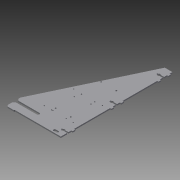
# Autodesk Inventor part: side_frame
Saved by Autodesk Inventor 2013 (Build 170138000, 138)
## iProperties
Created: 2013-11-17
Part Number: side_frame
Material: Generic
Document SubType Name: Modeling
Designer: Masta
Density: 1 g/cm^3
Author: Masta
Autodesk Inventor part; units mm, degrees
ref_plane "YZ Plane" through (0, 0, 0) normal (1, 0, 0) x (0, 1, 0)
ref_plane "XZ Plane" through (0, 0, 0) normal (0, 1, 0) x (-1, 0, 0)
ref_plane "XY Plane" through (0, 0, 0) normal (0, 0, 1) x (1, 0, 0)
sketch "Sketch1" plane through (0, 0, 0) normal (0, 0, 1) x (1, 0, 0)
  line L0 (255.7808, 350.0828) -> (255.7808, 358.8828)
  line L1 (251.6808, 67.29) -> (255.7808, 67.29)
  line L2 (255.7808, 67.29) -> (255.7808, 76.09)
  line L3 (255.7808, 76.09) -> (251.6808, 76.09)
  line L4 (251.6808, 76.09) -> (251.6808, 194.9901)
  line L5 (251.6808, 32.5401) -> (100.8808, 32.5401)
  line L6 (220.9195, 43.3685) -> (221.7479, 44.0042)
  line L7 (220.2838, 42.5401) -> (220.9195, 43.3685)
  line L8 (231.7439, 44.5401) -> (223.7479, 44.5401)
  line L9 (151.0808, 64.3506) -> (151.992, 63.6514)
  line L10 (230.5808, 213.3401) -> (234.5808, 213.3401)
  line L11 (150.0196, 64.7902) -> (151.0808, 64.3506)
  line L12 (234.5808, 211.5401) -> (239.6808, 211.5401)
  line L13 (233.7439, 44.0042) -> (234.5723, 43.3685)
  line L14 (251.6808, 57.7345) -> (239.6808, 57.7345)
  line L15 (239.6808, 57.7345) -> (239.6808, 59.5345)
  line L16 (230.5808, 53.3345) -> (234.5808, 53.3345)
  line L17 (234.5808, 51.5345) -> (239.6808, 51.5345)
  line L18 (239.6808, 59.5345) -> (234.5808, 59.5345)
  line L19 (234.5808, 53.3345) -> (234.5808, 51.5345)
  line L20 (239.6808, 53.3345) -> (251.6808, 53.3345)
  line L21 (239.6808, 51.5345) -> (239.6808, 53.3345)
  line L22 (251.6808, 57.7345) -> (251.6808, 67.29)
  line L23 (220.9195, 37.7117) -> (220.2838, 38.5401)
  line L24 (221.7479, 37.076) -> (220.9195, 37.7117)
  line L25 (222.7126, 36.6764) -> (221.7479, 37.076)
  line L26 (251.6808, 217.7401) -> (239.6808, 217.7401)
  line L27 (233.7439, 37.076) -> (232.7791, 36.6764)
  line L28 (232.7791, 36.6764) -> (231.7439, 36.5401)
  line L29 (235.6076, 39.5048) -> (235.208, 38.5401)
  line L30 (151.0808, 56.7296) -> (150.0196, 56.29)
  line L31 (255.7808, 236.0901) -> (251.6808, 236.0901)
  line L32 (251.6808, 236.0901) -> (251.6808, 350.0828)
  line L33 (255.7808, 203.7901) -> (251.6808, 203.7901)
  line L34 (251.6808, 194.9901) -> (255.7808, 194.9901)
  line L35 (255.7808, 194.9901) -> (255.7808, 203.7901)
  line L36 (251.6808, 227.2901) -> (251.6808, 217.7401)
  line L37 (251.6808, 213.3401) -> (251.6808, 203.7901)
  line L38 (251.6808, 382.3828) -> (255.7808, 382.3828)
  line L39 (255.7808, 382.3828) -> (255.7808, 391.1828)
  line L40 (255.7808, 391.1828) -> (251.6808, 391.1828)
  line L41 (251.6808, 391.1828) -> (251.6808, 400.5401)
  line L42 (255.7808, 358.8828) -> (251.6808, 358.8828)
  line L43 (251.6808, 350.0828) -> (255.7808, 350.0828)
  line L44 (73.8808, 35.5401) -> (73.8808, 51.1401)
  line L45 (235.208, 42.5401) -> (235.6076, 41.5754)
  line L46 (235.7439, 40.5401) -> (235.6076, 39.5048)
  line L47 (232.7791, 44.4038) -> (233.7439, 44.0042)
  line L48 (239.6808, 211.5401) -> (239.6808, 213.3401)
  line L49 (230.5808, 217.7401) -> (230.5808, 213.3401)
  line L50 (73.8808, 77.5401) -> (226.2808, 400.5401)
  line L51 (234.5808, 217.7401) -> (230.5808, 217.7401)
  line L52 (234.5808, 217.7401) -> (234.5808, 219.5401)
  line L53 (222.7126, 44.4038) -> (223.7479, 44.5401)
  line L54 (251.6808, 400.5401) -> (226.2808, 400.5401)
  line L55 (148.8808, 64.9401) -> (150.0196, 64.7902)
  line L56 (220.2838, 38.5401) -> (219.8842, 39.5048)
  line L57 (239.6808, 213.3401) -> (251.6808, 213.3401)
  line L58 (153.1308, 59.4013) -> (152.6913, 58.3401)
  line L59 (231.7439, 44.5401) -> (232.7791, 44.4038)
  line L60 (223.681, 36.5401) -> (222.7126, 36.6764)
  line L61 (231.7439, 36.5401) -> (223.681, 36.5401)
  line L62 (151.992, 63.6514) -> (152.6913, 62.7401)
  line L63 (153.2808, 60.5401) -> (153.1308, 59.4013)
  line L64 (239.6808, 219.5401) -> (234.5808, 219.5401)
  line L65 (98.8808, 30.5401) -> (78.8808, 30.5401)
  line L66 (152.6913, 58.3401) -> (151.992, 57.4288)
  line L67 (234.5808, 213.3401) -> (234.5808, 211.5401)
  line L68 (230.5808, 372.825) -> (230.5808, 368.425)
  line L69 (234.5808, 372.825) -> (230.5808, 372.825)
  line L70 (234.5808, 372.825) -> (234.5808, 374.625)
  line L71 (251.6808, 372.825) -> (239.6808, 372.825)
  line L72 (230.5808, 368.425) -> (234.5808, 368.425)
  line L73 (239.6808, 368.425) -> (251.6808, 368.425)
  line L74 (234.5808, 366.625) -> (239.6808, 366.625)
  line L75 (239.6808, 374.625) -> (234.5808, 374.625)
  line L76 (234.5808, 368.425) -> (234.5808, 366.625)
  line L77 (251.6808, 372.825) -> (251.6808, 382.3828)
  line L78 (251.6808, 368.425) -> (251.6808, 358.8828)
  line L79 (230.5808, 57.7345) -> (230.5808, 53.3345)
  line L80 (234.5808, 57.7345) -> (230.5808, 57.7345)
  line L81 (234.5808, 57.7345) -> (234.5808, 59.5345)
  line L82 (239.6808, 366.625) -> (239.6808, 368.425)
  line L83 (239.6808, 372.825) -> (239.6808, 374.625)
  line L84 (151.992, 57.4288) -> (151.0808, 56.7296)
  line L85 (219.7479, 40.5401) -> (219.8842, 41.5754)
  line L86 (221.7479, 44.0042) -> (222.7126, 44.4038)
  line L87 (78.8808, 56.1401) -> (148.8808, 56.1401)
  line L88 (78.8808, 56.1401) -> (73.8808, 51.1401)
  line L89 (78.8808, 64.9401) -> (148.8808, 64.9401)
  line L90 (73.8808, 69.9401) -> (73.8808, 77.5401)
  line L91 (78.8808, 64.9401) -> (73.8808, 69.9401)
  line L92 (251.6808, 227.2901) -> (255.7808, 227.2901)
  line L93 (255.7808, 227.2901) -> (255.7808, 236.0901)
  line L94 (234.5723, 43.3685) -> (235.208, 42.5401)
  line L95 (234.5723, 37.7117) -> (233.7439, 37.076)
  line L96 (152.6913, 62.7401) -> (153.1308, 61.6789)
  line L97 (153.1308, 61.6789) -> (153.2808, 60.5401)
  line L98 (219.8842, 41.5754) -> (220.2838, 42.5401)
  line L99 (239.6808, 217.7401) -> (239.6808, 219.5401)
  line L100 (78.8808, 30.5401) -> (73.8808, 35.5401)
  line L101 (100.8808, 32.5401) -> (98.8808, 30.5401)
  line L102 (235.6076, 41.5754) -> (235.7439, 40.5401)
  line L103 (235.208, 38.5401) -> (234.5723, 37.7117)
  line L104 (219.8842, 39.5048) -> (219.7479, 40.5401)
  line L105 (251.6808, 32.5401) -> (251.6808, 53.3345)
  line L106 (150.0196, 56.29) -> (148.8808, 56.1401)
  line L107 (136.6808, 189.5401) -> (231.6808, 189.5401) construction
  line L108 (231.6808, 189.5401) -> (231.6808, 93.5401) construction
  line L109 (231.6808, 93.5401) -> (136.6808, 93.5401) construction
  line L110 (136.6808, 93.5401) -> (136.6808, 189.5401) construction
  line L111 (164.6808, 93.5401) -> (208.6808, 93.5401) construction
  line L112 (208.6808, 93.5401) -> (208.6808, 187.5401) construction
  line L113 (208.6808, 187.5401) -> (164.6808, 187.5401) construction
  line L114 (164.6808, 187.5401) -> (164.6808, 93.5401) construction
  line L115 (160.3808, 93.5401) -> (208.6808, 93.5401) construction
  line L116 (208.6808, 93.5401) -> (208.6808, 168.5401) construction
  line L117 (208.6808, 168.5401) -> (160.3808, 168.5401) construction
  line L118 (160.3808, 168.5401) -> (160.3808, 93.5401) construction
  line L119 (208.6808, 168.5401) -> (208.6808, 174.8401) construction
  point P0 (0, 0)
  dimension "d0" = 177.8
  dimension "d9" = 95
  dimension "d10" = 96
  dimension "d11" = 44
  dimension "d12" = 94
  dimension "d15" = 48.3
  dimension "d16" = 75
  dimension "d18" = 6.3
  dimension "d19" = 23
  dimension "d20" = 20
  dimension "d21" = 63
  dimension "d22" = 4.1
  dimension "d23" = 8.8
  constraints: 240 end point, 17 collinear, 11 coincident, 7 parallel, 4 horizontal, 3 perpendicular, 1 vertical
  measures "d0" distance between parallel lines of L44 L105
  measures "d9" distance of L108.end L109.end
  measures "d10" distance of L107.end L108.end
  measures "d11" distance of L113.end L112.end
  measures "d12" distance of L111.end L112.end
  measures "d15" distance of L117.end L116.end
  measures "d16" distance of L116.end L111.end
  measures "d18" distance of L116.end L119.end
  measures "d19" distance between parallel lines of L108 L116
  measures "d20" distance between parallel lines of L4 L108
  measures "d21" distance between parallel lines of L65 L109
  measures "d22" distance between parallel lines of L2 L22
  measures "d23" distance of L1.end L2.end
extrude "Extrusion1" add sketch "Sketch1" against normal blind 4
hole "Hole1" at (136.6808, 189.5401, 0) at (136.6808, 93.5401, 0) at (231.6808, 93.5401, 0) at (231.6808, 189.5401, 0) at (160.3808, 93.5401, 0) at (208.6808, 93.5401, 0) at (208.6808, 174.8401, 0) at (160.3808, 168.5401, 0) at (164.6808, 93.5401, 0) at (164.6808, 187.5401, 0) at (208.6808, 187.5401, 0) direction (0, 0, -1) diameter 3.6 end through all
sketch "Sketch2" plane through (0, 0, 0) normal (0, 0, 1) x (1, 0, 0)
  line L0 (78.8808, 64.9401) -> (148.8808, 64.9401) projected
  line L1 (251.6808, 76.09) -> (251.6808, 194.9901) projected
  line L2 (162.1808, 104.9401) -> (212.1808, 104.9401) construction
  line L3 (212.1808, 104.9401) -> (212.1808, 254.9401) construction
  line L4 (212.1808, 254.9401) -> (162.1808, 254.9401) construction
  line L5 (162.1808, 254.9401) -> (162.1808, 104.9401) construction
  line L6 (162.1808, 104.9401) -> (212.1808, 254.9401) construction
  line L7 (212.1808, 104.9401) -> (162.1808, 254.9401) construction
  line L8 (129.6808, 69.9401) -> (244.6808, 69.9401) construction
  line L9 (244.6808, 69.9401) -> (244.6808, 289.9401) construction
  line L10 (244.6808, 289.9401) -> (129.6808, 289.9401) construction
  line L11 (129.6808, 289.9401) -> (129.6808, 69.9401) construction
  line L12 (129.6808, 69.9401) -> (244.6808, 289.9401) construction
  line L13 (244.6808, 69.9401) -> (129.6808, 289.9401) construction
  point P0 (0, 0)
  point P1 (187.1808, 179.9401)
  point P2 (187.1808, 179.9401)
  dimension "d33" = 50
  dimension "d34" = 150
  dimension "d35" = 115
  dimension "d36" = 220
  dimension "d37" = 5
  dimension "d38" = 7
  constraints: 24 end point, 5 midpoint, 4 coincident, 4 parallel, 2 horizontal, 2 perpendicular
  measures "d33" distance of L4.end L3.end
  measures "d34" distance of L3.end L2.end
  measures "d35" distance of L10.end L9.end
  measures "d36" distance of L9.end L8.end
  measures "d37" distance between parallel lines of L8 L0
  measures "d38" distance between parallel lines of L1 L9
hole "Hole2" at (162.1808, 254.9401, 0) at (162.1808, 104.9401, 0) at (212.1808, 104.9401, 0) at (212.1808, 254.9401, 0) direction (0, 0, -1) diameter 4.6 end through all
body "Solid1"
